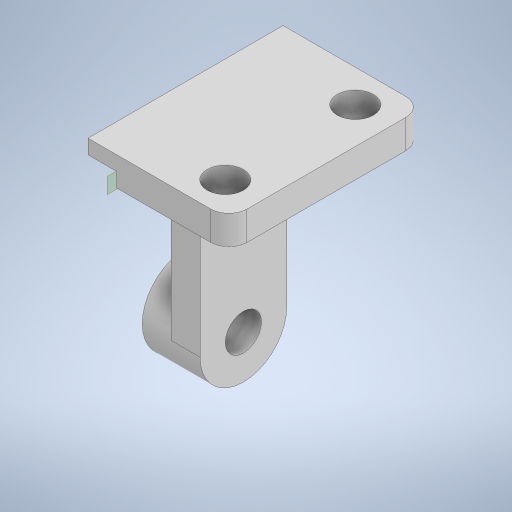
# Autodesk Inventor part: yatak
Saved by Autodesk Inventor 2024 (Build 280153000, 153)
## iProperties
Created: 2024-06-04
Part Number: yatak
Material: Generic
Document SubType Name: Modeling
Designer: Ricsi
Density: 1 g/cm^3
Appearance: Default
Author: Ricsi
Autodesk Inventor part; units mm, degrees
ref_plane "YZ Plane" through (0, 0, 0) normal (1, 0, 0) x (0, 1, 0)
ref_plane "XZ Plane" through (0, 0, 0) normal (0, 1, 0) x (-1, 0, 0)
ref_plane "XY Plane" through (0, 0, 0) normal (0, 0, 1) x (1, 0, 0)
sketch "Sketch1" plane through (0, 0, 0) normal (0, 1, 0) x (-1, 0, 0)
  line L0 (6.6946, 16.8791) -> (-27.3054, 16.8791)
  line L1 (-32.3054, 11.8791) -> (-32.3054, -32.1209)
  line L2 (-27.3054, -37.1209) -> (6.6946, -37.1209)
  line L3 (6.6946, -37.1209) -> (6.6946, 16.8791)
  arc A0 (-27.3054, 16.8791) -> (-32.3054, 11.8791) centre (-27.3054, 11.8791) ccw
  arc A1 (-32.3054, -32.1209) -> (-27.3054, -37.1209) centre (-27.3054, -32.1209) ccw
  circle A2 centre (-22.3054, 7.8791) radius 5
  circle A3 centre (-22.3054, -28.1209) radius 5
  point P0 (0, 0)
  point P1 (-32.3054, -37.1209)
  point P2 (-32.3054, 16.8791)
  dimension "d0" = 39
  dimension "d1" = 54
  dimension "d2" = 5
  dimension "d3" = 5
  dimension "d5" = 10
  dimension "d6" = 10
  dimension "d7" = 9
  dimension "d8" = 9
  constraints: 8 end point, 4 centre point, 4 point on circle, 4 point on line, 4 tangent, 2 parallel, 1 horizontal, 1 perpendicular
  measures "d0" distance of L2.end point (-32.305, -37.121)
  measures "d1" distance of point (-32.305, -37.121) point (-32.305, 16.879)
  measures "d2" radius of A0
  measures "d3" radius of A1
  measures "d5" diameter of A2
  measures "d6" diameter of A3
  measures "d7" distance from line of L0 A2.centre
  measures "d8" distance from line of A3.centre L2
extrude "Extrusion1" add sketch "Sketch1" along normal blind 8
sketch "Sketch2" plane through (0, 0, 0) normal (0, -1, 0) x (1, 0, 0)
  line L0 (-6.6946, -37.1209) -> (-6.6946, 16.8791) projected
  line L1 (-6.6946, 16.8791) -> (1.3054, 16.8791)
  line L2 (-6.6946, 16.8791) -> (27.3054, 16.8791) projected
  line L3 (1.3054, 16.8791) -> (1.3054, -37.1209)
  line L4 (27.3054, -37.1209) -> (-6.6946, -37.1209) projected
  line L5 (-6.6946, -37.1209) -> (1.3054, -37.1209)
  line L6 (-6.6946, -37.1209) -> (-6.6946, 16.8791)
  point P0 (0, 0)
  dimension "d11" = 8
  constraints: 8 end point, 2 collinear, 2 point on line, 1 vertical
  measures "d11" distance of L0.end L1.end
extrude "Extrusion2" cut sketch "Sketch2" against normal blind 4
ref_plane "Work Plane1" through (1.3054, 0, -37.1209) normal (-1, 0, 0) x (0, 0, 1)
sketch "Sketch3" plane through (1.3054, 0, -37.1209) normal (-1, 0, 0) x (0, 0, 1)
  line L0 (54, 0) -> (54, 8) projected
  circle A0 centre (27, -44) radius 5
  arc A1 (15, -44) -> (39, -44) centre (27, -44) ccw
  line L1 (39, -44) -> (39, 0)
  line L2 (49, 0) -> (5, 0) projected
  line L3 (15, -44) -> (15, 0)
  line L4 (39, 0) -> (15, 0)
  point P0 (37.1209, 0)
  dimension "d17" = 10
  dimension "d18" = 24
  constraints: 6 end point, 2 centre point, 2 point on circle, 2 point on line, 1 coincident, 1 collinear, 1 parallel, 1 vertical
  measures "d17" diameter of A0
  measures "d18" diameter of A1
extrude "Extrusion3" add sketch "Sketch3" against normal blind 8
sketch "Sketch4" plane through (1.3054, 0, 16.8791) normal (-1, 0, 0) x (0, 0, 1)
  line L0 (0, 4) -> (0, 0) projected
  circle A0 centre (-27, -44) radius 12
  point P0 (-16.8791, 0)
  dimension "d23" = 24
  constraints: 1 centre point
  measures "d23" diameter of A0
extrude "Extrusion4" add sketch "Sketch4" along normal blind 8
sketch "Sketch5" plane through (-6.6946, -44, -10.1209) normal (-1, 0, 0) x (0, 0, 1)
  circle A0 centre (0, 0) radius 5
  point P0 (10.1209, 44)
  dimension "d26" = 10
  constraints: 1 centre point
  measures "d26" diameter of A0
extrude "Extrusion5" cut sketch "Sketch5" against normal blind 8
fillet "Face Fillet1" radius 5 1 edges at (5.3054, 0, 1.8791)
fillet "Face Fillet2" radius 5 1 edges at (5.3054, 0, -22.1209)
body "Solid1"
